Autodesk Fusion 360 part; units mm, degrees
note: some values were not read from the file. Chosen so that the rebuilt part matches the saved one: which bodies a step acts on; which pieces of a blend or face edit are solid. Set by a fixed rule: which sketch regions a step uses.
(part 2 of 2)
sketch "outline" plane through (0, 0, 0) normal (0, 0, 1) x (1, 0, 0)
  line L0 (16.3638, 40.64) -> (-16.3638, 40.64)
  line L1 (-40.64, 16.3638) -> (-40.64, -16.3638)
  line L2 (-16.3638, -40.64) -> (16.3638, -40.64)
  line L3 (40.64, -16.3638) -> (40.64, 16.3638)
  circle A0 centre (16.129, 37.719) radius 1.5
  circle A1 centre (-37.719, 16.129) radius 1.5
  circle A2 centre (-16.129, -37.719) radius 1.5
  circle A3 centre (37.719, -16.129) radius 1.5
  circle A4 centre (37.719, 16.129) radius 1.5
  circle A5 centre (-16.129, 37.719) radius 1.5
  circle A6 centre (-37.719, -16.129) radius 1.5
  circle A7 centre (16.129, -37.719) radius 1.5
  line L4 (-18.1316, 39.9078) -> (-39.9078, 18.1316)
  line L5 (-39.9078, -18.1316) -> (-18.1316, -39.9078)
  line L6 (18.1316, -39.9078) -> (39.9078, -18.1316)
  line L7 (39.9078, 18.1316) -> (18.1316, 39.9078)
  arc A8 (18.1316, 39.9078) -> (16.3638, 40.64) centre (16.3638, 38.14) ccw
  arc A9 (40.64, 16.3638) -> (39.9078, 18.1316) centre (38.14, 16.3638) ccw
  arc A10 (39.9078, -18.1316) -> (40.64, -16.3638) centre (38.14, -16.3638) ccw
  arc A11 (-40.64, -16.3638) -> (-39.9078, -18.1316) centre (-38.14, -16.3638) ccw
  arc A12 (-18.1316, -39.9078) -> (-16.3638, -40.64) centre (-16.3638, -38.14) ccw
  arc A13 (-16.3638, 40.64) -> (-18.1316, 39.9078) centre (-16.3638, 38.14) ccw
  arc A14 (-39.9078, 18.1316) -> (-40.64, 16.3638) centre (-38.14, 16.3638) ccw
  arc A15 (16.3638, -40.64) -> (18.1316, -39.9078) centre (16.3638, -38.14) ccw
  dimension "d2" = 40.64
  dimension "d3" = 3
  dimension "d4" = 16.129
  dimension "d5" = 37.719
  dimension "d7" = 360
  dimension "d8" = 3
  dimension "d9" = 16.129
  dimension "d10" = 37.719
  dimension "d12" = 360
  dimension "d14" = 2.5
  dimension "d15" = 2.5
  dimension "d16" = 2.5
  dimension "d17" = 2.5
  dimension "d18" = 2.5
  dimension "d19" = 2.5
  dimension "d20" = 2.5
  dimension "d23" = 2.5
  measures "d2" distance of origin L3
  measures "d3" diameter of A0
  measures "d4" distance of origin A0.centre
  measures "d5" distance of origin A0.centre
  measures "d8" diameter of A4
  measures "d9" distance of origin A4.centre
  measures "d10" distance of origin A4.centre
  measures "d14" radius of A8
  measures "d15" radius of A9
  measures "d16" radius of A10
  measures "d17" radius of A11
  measures "d18" radius of A12
  measures "d19" radius of A13
  measures "d20" radius of A14
  measures "d23" radius of A15
extrude "Extrude1" add sketch "outline" along normal blind 1.6 makes body 1
extrude "Extrude2" cut sketch "cpx crickit" along normal up to surface (1.6 mm away) contours A88 | A89 | A90 | A91 | A92 | A93 | A94 | A95 | A96 | A97 | A98 | A99 | A100 | A101 | A102 | A103 | A104 | A105 | A106 | A107 | A108 | A109 | A110 | A111 | A112 | A113 | A114 | A115 | A116 | A117 | A118 | A119 | A120 | A121 | A122 | A123 | A124 | A125 | A126 | A127 | A128 | A129 | A130 | A131 | A132 | A133 | A134 | A135 | A136 | A137 | A138 | A139 | A140 | A141 | A142 | A143 | A144 | A145 | A146 | A147 | A148 bodies 1
sketch "PCB" plane through (0, 0, 1.6) normal (0, 0, 1) x (-1, 0, 0)
  circle A0 centre (-26.1731, -21.2233) radius 0.635
  circle A1 centre (11.6332, -20.066) radius 1.5
  circle A2 centre (24.5963, -22.8001) radius 0.635
  circle A3 centre (19.2081, -24.5962) radius 0.635
  circle A4 centre (22.8002, -21.0041) radius 0.635
  circle A5 centre (33.528, 3.81) radius 0.635
  circle A6 centre (36.068, -1.27) radius 0.635
  circle A7 centre (33.528, -6.35) radius 0.635
  circle A8 centre (36.068, -8.89) radius 0.635
  circle A9 centre (30.988, -1.27) radius 0.635
  circle A10 centre (33.528, -8.89) radius 0.635
  circle A11 centre (-33.528, 0) radius 0.635
  circle A12 centre (-30.2288, 18.0312) radius 0.635
  circle A13 centre (-22.7949, 25.4651) radius 0.635
  circle A14 centre (24.8067, 29.5692) radius 1.5
  circle A15 centre (29.3787, 24.9972) radius 1.5
  circle A16 centre (-11.6332, 20.066) radius 1.5
  circle A17 centre (-27.7539, 20.5061) radius 0.635
  circle A18 centre (-33.528, 3.5) radius 0.635
  circle A19 centre (33.528, -1.27) radius 0.635
  circle A20 centre (36.068, 3.81) radius 0.635
  circle A21 centre (30.988, -6.35) radius 0.635
  circle A22 centre (30.988, 6.35) radius 0.635
  circle A23 centre (33.528, -3.81) radius 0.635
  circle A24 centre (36.068, -6.35) radius 0.635
  circle A25 centre (24.5963, -19.208) radius 0.635
  circle A26 centre (24.5963, -26.3922) radius 0.635
  circle A27 centre (22.8002, -24.5962) radius 0.635
  circle A28 centre (17.78, -14.859) radius 1.5
  circle A29 centre (-28.6479, -18.7485) radius 0.635
  circle A30 centre (-18.7485, -28.6479) radius 0.635
  circle A31 centre (21.844, -7.9248) radius 1.5
  circle A32 centre (21.0041, -22.8001) radius 0.635
  circle A33 centre (26.3923, -24.5962) radius 0.635
  circle A34 centre (26.3923, -21.0041) radius 0.635
  circle A35 centre (30.988, -3.81) radius 0.635
  circle A36 centre (30.988, 1.27) radius 0.635
  circle A37 centre (33.528, 8.89) radius 0.635
  circle A38 centre (36.068, 8.89) radius 0.635
  circle A39 centre (30.988, 8.89) radius 0.635
  circle A40 centre (36.068, 1.27) radius 0.635
  circle A41 centre (-33.528, -3.5) radius 0.635
  circle A42 centre (-21.844, 7.9248) radius 1.5
  circle A43 centre (-20.32, 27.94) radius 0.635
  circle A44 centre (20.1077, 34.2682) radius 1.5
  circle A45 centre (34.1412, 20.2982) radius 1.5
  circle A46 centre (-17.8451, 30.4149) radius 0.635
  circle A47 centre (-17.78, 14.859) radius 1.5
  circle A48 centre (-33.528, 7) radius 0.635
  circle A49 centre (-33.528, -7) radius 0.635
  circle A50 centre (30.988, -8.89) radius 0.635
  circle A51 centre (30.988, 3.81) radius 0.635
  circle A52 centre (33.528, 1.27) radius 0.635
  circle A53 centre (36.068, 6.35) radius 0.635
  circle A54 centre (33.528, 6.35) radius 0.635
  circle A55 centre (36.068, -3.81) radius 0.635
  circle A56 centre (22.8002, -28.1883) radius 0.635
  circle A57 centre (21.0041, -26.3922) radius 0.635
  circle A58 centre (28.1884, -22.8001) radius 0.635
  circle A59 centre (-21.2233, -26.1731) radius 0.635
  circle A60 centre (-23.6982, -23.6982) radius 0.635
  circle A61 centre (-16.129, -37.719) radius 1.5
  circle A62 centre (-16.129, 37.719) radius 1.5
  circle A63 centre (16.129, 37.719) radius 1.5
  circle A64 centre (-37.719, 16.129) radius 1.5
  circle A65 centre (16.129, -37.719) radius 1.5
  circle A66 centre (-37.719, -16.129) radius 1.5
  circle A67 centre (37.719, 16.129) radius 1.5
  circle A68 centre (37.719, -16.129) radius 1.5
  arc A69 (-16.3638, 40.64) -> (-18.1316, 39.9078) centre (-16.3638, 38.14) ccw
  line L0 (-18.1316, 39.9078) -> (-39.9078, 18.1316)
  arc A70 (-39.9078, 18.1316) -> (-40.64, 16.3638) centre (-38.14, 16.3638) ccw
  line L1 (-40.64, 16.3638) -> (-40.64, -16.3638)
  arc A71 (-40.64, -16.3638) -> (-39.9078, -18.1316) centre (-38.14, -16.3638) ccw
  line L2 (-39.9078, -18.1316) -> (-18.1316, -39.9078)
  arc A72 (-18.1316, -39.9078) -> (-16.3638, -40.64) centre (-16.3638, -38.14) ccw
  line L3 (-16.3638, -40.64) -> (16.3638, -40.64)
  arc A73 (16.3638, -40.64) -> (18.1316, -39.9078) centre (16.3638, -38.14) ccw
  line L4 (18.1316, -39.9078) -> (39.9078, -18.1316)
  arc A74 (39.9078, -18.1316) -> (40.64, -16.3638) centre (38.14, -16.3638) ccw
  line L5 (40.64, -16.3638) -> (40.64, 16.3638)
  arc A75 (40.64, 16.3638) -> (39.9078, 18.1316) centre (38.14, 16.3638) ccw
  line L6 (39.9078, 18.1316) -> (18.1316, 39.9078)
  arc A76 (18.1316, 39.9078) -> (16.3638, 40.64) centre (16.3638, 38.14) ccw
  line L7 (16.3638, 40.64) -> (-16.3638, 40.64)
  line L8 (37.518, -10.34) -> (29.538, -10.34)
  line L9 (29.538, -10.34) -> (29.538, 10.34)
  line L10 (29.538, 10.34) -> (37.518, 10.34)
  line L11 (37.518, 10.34) -> (37.518, -10.34)
  line L12 (22.8002, -29.9844) -> (29.9844, -22.8001)
  line L13 (29.9844, -22.8001) -> (24.5963, -17.412)
  line L14 (24.5963, -17.412) -> (17.412, -24.5962)
  line L15 (17.412, -24.5962) -> (22.8002, -29.9844)
  line L16 (24.5963, -28.1883) -> (19.2081, -22.8001)
  line L17 (26.3923, -26.3922) -> (21.0041, -21.0041)
  line L18 (28.1884, -24.5962) -> (22.8002, -19.208)
  line L19 (-3.8, 40.64) -> (3.8, 40.64)
  line L20 (3.8, 40.64) -> (3.8, 35.04)
  line L21 (3.8, 35.04) -> (-3.8, 35.04)
  line L22 (-3.8, 35.04) -> (-3.8, 40.64)
  line L23 (-3.8, 40.64) -> (3.8, 35.04) construction
  line L24 (3.8, 40.64) -> (-3.8, 35.04) construction
  line L25 (0, 37.84) -> (0, 40.64) construction
  line L26 (6.505, 39.4055) -> (10.005, 39.4055)
  line L27 (10.005, 39.4055) -> (10.005, 35.9055)
  line L28 (10.005, 35.9055) -> (6.505, 35.9055)
  line L29 (6.505, 35.9055) -> (6.505, 39.4055)
  line L30 (6.505, 39.4055) -> (10.005, 35.9055) construction
  line L31 (10.005, 39.4055) -> (6.505, 35.9055) construction
  line L32 (3.865, -29.74) -> (-5.135, -29.74)
  line L33 (-5.135, -29.74) -> (-5.135, -44.14)
  line L34 (-5.135, -44.14) -> (3.865, -44.14)
  line L35 (3.865, -44.14) -> (3.865, -29.74)
  line L36 (3.865, -29.74) -> (-5.135, -44.14) construction
  line L37 (-5.135, -29.74) -> (3.865, -44.14) construction
  line L38 (-12.017, -33.195) -> (-6.017, -33.195)
  line L39 (-6.017, -33.195) -> (-6.017, -39.195)
  line L40 (-6.017, -39.195) -> (-12.017, -39.195)
  line L41 (-12.017, -39.195) -> (-12.017, -33.195)
  line L42 (-12.017, -33.195) -> (-6.017, -39.195) construction
  line L43 (-6.017, -33.195) -> (-12.017, -39.195) construction
  circle A77 centre (-9.017, -36.195) radius 1.5
  line L44 (8.029, -31.679) -> (11.529, -31.679)
  line L45 (11.529, -31.679) -> (11.529, -38.679)
  line L46 (11.529, -38.679) -> (8.029, -38.679)
  line L47 (8.029, -38.679) -> (8.029, -31.679)
  line L48 (8.029, -31.679) -> (11.529, -38.679) construction
  line L49 (11.529, -31.679) -> (8.029, -38.679) construction
  line L50 (15.6765, -27.19) -> (14.6765, -27.19)
  line L51 (14.6765, -27.19) -> (14.6765, -28.69)
  line L52 (14.6765, -28.69) -> (15.6765, -28.69)
  line L53 (15.6765, -28.69) -> (15.6765, -27.19)
  line L54 (15.6765, -27.19) -> (14.6765, -28.69) construction
  line L55 (14.6765, -27.19) -> (15.6765, -28.69) construction
  line L56 (13.2635, -27.19) -> (12.2635, -27.19)
  line L57 (12.2635, -27.19) -> (12.2635, -28.69)
  line L58 (12.2635, -28.69) -> (13.2635, -28.69)
  line L59 (13.2635, -28.69) -> (13.2635, -27.19)
  line L60 (13.2635, -27.19) -> (12.2635, -28.69) construction
  line L61 (12.2635, -27.19) -> (13.2635, -28.69) construction
  line L62 (31.369, -14.7236) -> (35.1874, -18.542)
  line L63 (35.1874, -18.542) -> (31.369, -22.3604)
  line L64 (31.369, -22.3604) -> (27.5506, -18.542)
  line L65 (27.5506, -18.542) -> (31.369, -14.7236)
  line L66 (31.369, -14.7236) -> (31.369, -22.3604) construction
  line L67 (35.1874, -18.542) -> (27.5506, -18.542) construction
  circle A78 centre (31.369, -18.542) radius 2.5
  line L68 (-34.577, -9.746) -> (-29.177, -9.746)
  line L69 (-29.177, -9.746) -> (-29.177, -15.146)
  line L70 (-29.177, -15.146) -> (-34.577, -15.146)
  line L71 (-34.577, -15.146) -> (-34.577, -9.746)
  line L72 (-34.577, -9.746) -> (-29.177, -15.146) construction
  line L73 (-29.177, -9.746) -> (-34.577, -15.146) construction
  circle A79 centre (-31.877, -12.446) radius 2.5
  line L74 (-30.128, -9) -> (-36.928, -9)
  line L75 (-36.928, -9) -> (-36.928, 9)
  line L76 (-36.928, 9) -> (-30.128, 9)
  line L77 (-30.128, 9) -> (-30.128, -9)
  line L78 (-19.7384, -32.4663) -> (-32.4664, -19.7384)
  line L79 (-32.4664, -19.7384) -> (-27.658, -14.93)
  line L80 (-27.658, -14.93) -> (-14.9301, -27.658)
  line L81 (-14.9301, -27.658) -> (-19.7384, -32.4663)
  line L82 (-21.805, 21.6467) -> (-26.6133, 26.455)
  line L83 (-26.6133, 26.455) -> (-18.8351, 34.2332)
  line L84 (-18.8351, 34.2332) -> (-14.0268, 29.4249)
  line L85 (-14.0268, 29.4249) -> (-21.805, 21.6467)
  line L86 (-24.2091, 24.0509) -> (-16.4309, 31.8291) construction
  line L87 (-29.2389, 14.2128) -> (-23.9355, 19.5161)
  line L88 (-23.9355, 19.5161) -> (-28.7439, 24.3245)
  line L89 (-28.7439, 24.3245) -> (-34.0472, 19.0211)
  line L90 (-34.0472, 19.0211) -> (-29.2389, 14.2128)
  circle A80 centre (-20.141, 20.194) radius 1.5
  line L91 (-3.5, 29.154) -> (3.5, 29.154)
  line L92 (3.5, 29.154) -> (3.5, 22.154)
  line L93 (3.5, 22.154) -> (-3.5, 22.154)
  line L94 (-3.5, 22.154) -> (-3.5, 29.154)
  line L95 (-3.5, 29.154) -> (3.5, 22.154) construction
  line L96 (3.5, 29.154) -> (-3.5, 22.154) construction
  line L97 (-18.456, 4.659) -> (-14.056, 4.659)
  line L98 (-14.056, 4.659) -> (-14.056, -0.341)
  line L99 (-14.056, -0.341) -> (-18.456, -0.341)
  line L100 (-18.456, -0.341) -> (-18.456, 4.659)
  line L101 (-18.456, 4.659) -> (-14.056, -0.341) construction
  line L102 (-14.056, 4.659) -> (-18.456, -0.341) construction
  line L103 (-17.3046, -9.9859) -> (-14.4762, -7.1575)
  line L104 (-14.4762, -7.1575) -> (-7.4051, -14.2286)
  line L105 (-7.4051, -14.2286) -> (-10.2336, -17.057)
  line L106 (-10.2336, -17.057) -> (-17.3046, -9.9859)
  line L107 (-17.3046, -9.9859) -> (-7.4051, -14.2286) construction
  line L108 (-14.4762, -7.1575) -> (-10.2336, -17.057) construction
  point P0 (0, 37.84)
  point P1 (8.255, 37.6555)
  point P2 (-0.635, -36.94)
  point P3 (-9.017, -36.195)
  point P4 (9.779, -35.179)
  point P5 (15.1765, -27.94)
  point P6 (12.7635, -27.94)
  point P7 (31.369, -18.542)
  point P8 (-31.877, -12.446)
  point P9 (0, 25.654)
  point P10 (-16.256, 2.159)
  point P11 (-12.3549, -12.1073)
  dimension "d61" = 1.45
  dimension "d62" = 1.45
  dimension "d63" = 1.45
  dimension "d64" = 1.45
  dimension "d81" = 90
  dimension "d82" = 90
  dimension "d83" = 1.27
  dimension "d84" = 1.27
  dimension "d88" = 2.54
  dimension "d89" = 0
  dimension "d90" = 1.27
  dimension "d91" = 1.27
  dimension "d92" = 1.27
  dimension "d110" = 7.6
  dimension "d111" = 5.6
  dimension "d117" = 3.5
  dimension "d118" = 3.5
  dimension "d119" = 8.255
  dimension "d120" = 37.6555
  dimension "d126" = 9
  dimension "d127" = 14.4
  dimension "d128" = 0.635
  dimension "d129" = 3.5
  dimension "d147" = 6
  dimension "d148" = 6
  dimension "d149" = 9.017
  dimension "d150" = 36.195
  dimension "d151" = 3
  dimension "d157" = 7
  dimension "d158" = 3.5
  dimension "d159" = 9.779
  dimension "d160" = 35.179
  dimension "d170" = 1.5
  dimension "d171" = 1
  dimension "d172" = 15.1765
  dimension "d173" = 27.94
  dimension "d174" = 1.5
  dimension "d175" = 1
  dimension "d176" = 12.7635
  dimension "d179" = 5.4
  dimension "d180" = 5.4
  dimension "d181" = 31.369
  dimension "d182" = 18.542
  dimension "d183" = 5
  dimension "d190" = 5.4
  dimension "d191" = 5.4
  dimension "d192" = 5
  dimension "d193" = 31.877
  dimension "d194" = 12.446
  dimension "d201" = 3.4
  dimension "d202" = 3.4
  dimension "d203" = 2
  dimension "d204" = 2
  dimension "d239" = 2
  dimension "d241" = 90
  dimension "d242" = 90
  dimension "d243" = 3.4
  dimension "d244" = 18
  dimension "d277" = 3.4
  dimension "d278" = 3.4
  dimension "d279" = 2
  dimension "d282" = 11
  dimension "d283" = 2
  dimension "d284" = 3.4
  dimension "d285" = 3.4
  dimension "d286" = 7.5
  dimension "d338" = 3
  dimension "d339" = 20.194
  dimension "d340" = 20.141
  dimension "d349" = 7
  dimension "d350" = 7
  dimension "d351" = 25.654
  dimension "d354" = 4.4
  dimension "d355" = 5
  dimension "d356" = 16.256
  dimension "d360" = 2.159
  dimension "d361" = 10
  dimension "d362" = 4
  dimension "d363" = 12.3549
  dimension "d364" = 12.1073
  measures "d61" distance of A8.centre L11
  measures "d62" distance of A8.centre L8
  measures "d63" distance of A50.centre L9
  measures "d64" distance of A39.centre L10
  measures "d81" angle of L12 L13
  measures "d82" angle of L13 L14
  measures "d83" distance of A58.centre L13
  measures "d84" distance of A58.centre L12
  measures "d90" distance of A56.centre L15
  measures "d91" distance of A57.centre L16
  measures "d92" distance of A3.centre L14
  measures "d110" distance of L20.end L21.end
  measures "d111" distance of L19.end L20.end
  measures "d117" distance of L27.end L28.end
  measures "d118" distance of L26.end L27.end
  measures "d119" distance of origin P1
  measures "d120" distance of origin P1
  measures "d126" distance of L33.end L34.end
  measures "d127" distance of L32.end L33.end
  measures "d128" distance of origin P2
  measures "d129" distance of L3 L34
  measures "d147" distance of L39.end L40.end
  measures "d148" distance of L38.end L39.end
  measures "d149" distance of origin P3
  measures "d150" distance of origin P3
  measures "d151" diameter of A77
  measures "d157" distance of L44.end L45.end
  measures "d158" distance of L45.end L46.end
  measures "d159" distance of origin P4
  measures "d160" distance of origin P4
  measures "d170" distance of L50.end L51.end
  measures "d171" distance of L51.end L52.end
  measures "d172" distance of origin P5
  measures "d173" distance of origin P5
  measures "d174" distance of L56.end L57.end
  measures "d175" distance of L57.end L58.end
  measures "d176" distance of origin P6
  measures "d179" distance of L62.end L63.end
  measures "d180" distance of L63.end L64.end
  measures "d181" distance of origin P7
  measures "d182" distance of origin P7
  measures "d183" diameter of A78
  measures "d190" distance of L69.end L70.end
  measures "d191" distance of L68.end L69.end
  measures "d192" diameter of A79
  measures "d193" distance of origin P8
  measures "d194" distance of origin P8
  measures "d201" distance of A48.centre L75
  measures "d202" distance of A48.centre L77
  measures "d203" distance of A48.centre L76
  measures "d204" distance of A49.centre L74
  measures "d239" distance of A30.centre L81
  measures "d241" angle of L78 L81
  measures "d242" angle of L79 L80
  measures "d243" distance of A30.centre L80
  measures "d244" distance of L78.start L78.end
  measures "d277" distance of A13.centre L83
  measures "d278" distance of A13.centre L85
  measures "d279" distance of A13.centre L82
  measures "d282" distance of L86.start L86.end
  measures "d283" distance of A12.centre L90
  measures "d284" distance of A12.centre L87
  measures "d285" distance of A12.centre L89
  measures "d286" distance of L87.start L87.end
  measures "d338" diameter of A80
  measures "d339" distance of origin A80.centre
  measures "d340" distance of origin A80.centre
  measures "d349" distance of L92.end L93.end
  measures "d350" distance of L91.end L92.end
  measures "d351" distance of origin P9
  measures "d354" distance of L98.end L99.end
  measures "d355" distance of L97.end L98.end
  measures "d356" distance of origin P10
  measures "d360" distance of origin P10
  measures "d361" distance of L103.end L104.end
  measures "d362" distance of L104.end L105.end
  measures "d363" distance of origin P11
  measures "d364" distance of origin P11
extrude "Extrude8" add sketch "PCB" along normal blind 1 separate body contours L26 L27 L28 L29 makes body 2
extrude "Extrude3" add sketch "PCB" along normal blind 8.6 separate body contours A5 | A6 | A7 | A8 | A9 | A10 | A19 | A20 | A21 | A22 | A23 | A24 | A35 | A36 | A37 | A38 | A39 | A40 | A50 | A51 | A52 | A53 | A54 | A55 | L8 L9 L10 L11 makes body 3
sketch "sio block" plane through (0, 0, 10.2) normal (0, 0, 1) x (-1, 0, 0)
  line L0 (37.518, 10.34) -> (29.538, 10.34)
  line L1 (29.538, 10.34) -> (29.538, -10.34)
  line L2 (29.538, -10.34) -> (37.518, -10.34)
  line L3 (37.518, -10.34) -> (37.518, 10.34)
  line L4 (35.768, -8.59) -> (36.368, -8.59)
  line L5 (36.368, -8.59) -> (36.368, -9.19)
  line L6 (36.368, -9.19) -> (35.768, -9.19)
  line L7 (35.768, -9.19) -> (35.768, -8.59)
  line L8 (35.768, -8.59) -> (36.368, -9.19) construction
  line L9 (36.368, -8.59) -> (35.768, -9.19) construction
  line L10 (33.828, -9.19) -> (33.228, -9.19)
  line L11 (33.228, -9.19) -> (33.228, -8.59)
  line L12 (33.228, -8.59) -> (33.828, -8.59)
  line L13 (33.828, -8.59) -> (33.828, -9.19)
  line L14 (31.288, -9.19) -> (30.688, -9.19)
  line L15 (30.688, -9.19) -> (30.688, -8.59)
  line L16 (30.688, -8.59) -> (31.288, -8.59)
  line L17 (31.288, -8.59) -> (31.288, -9.19)
  line L18 (36.368, -6.65) -> (35.768, -6.65)
  line L19 (35.768, -6.65) -> (35.768, -6.05)
  line L20 (35.768, -6.05) -> (36.368, -6.05)
  line L21 (36.368, -6.05) -> (36.368, -6.65)
  line L22 (33.828, -6.65) -> (33.228, -6.65)
  line L23 (33.228, -6.65) -> (33.228, -6.05)
  line L24 (33.228, -6.05) -> (33.828, -6.05)
  line L25 (33.828, -6.05) -> (33.828, -6.65)
  line L26 (31.288, -6.65) -> (30.688, -6.65)
  line L27 (30.688, -6.65) -> (30.688, -6.05)
  line L28 (30.688, -6.05) -> (31.288, -6.05)
  line L29 (31.288, -6.05) -> (31.288, -6.65)
  line L30 (36.368, -4.11) -> (35.768, -4.11)
  line L31 (35.768, -4.11) -> (35.768, -3.51)
  line L32 (35.768, -3.51) -> (36.368, -3.51)
  line L33 (36.368, -3.51) -> (36.368, -4.11)
  line L34 (33.828, -4.11) -> (33.228, -4.11)
  line L35 (33.228, -4.11) -> (33.228, -3.51)
  line L36 (33.228, -3.51) -> (33.828, -3.51)
  line L37 (33.828, -3.51) -> (33.828, -4.11)
  line L38 (31.288, -4.11) -> (30.688, -4.11)
  line L39 (30.688, -4.11) -> (30.688, -3.51)
  line L40 (30.688, -3.51) -> (31.288, -3.51)
  line L41 (31.288, -3.51) -> (31.288, -4.11)
  line L42 (36.368, -1.57) -> (35.768, -1.57)
  line L43 (35.768, -1.57) -> (35.768, -0.97)
  line L44 (35.768, -0.97) -> (36.368, -0.97)
  line L45 (36.368, -0.97) -> (36.368, -1.57)
  line L46 (33.828, -1.57) -> (33.228, -1.57)
  line L47 (33.228, -1.57) -> (33.228, -0.97)
  line L48 (33.228, -0.97) -> (33.828, -0.97)
  line L49 (33.828, -0.97) -> (33.828, -1.57)
  line L50 (31.288, -1.57) -> (30.688, -1.57)
  line L51 (30.688, -1.57) -> (30.688, -0.97)
  line L52 (30.688, -0.97) -> (31.288, -0.97)
  line L53 (31.288, -0.97) -> (31.288, -1.57)
  line L54 (36.368, 0.97) -> (35.768, 0.97)
  line L55 (35.768, 0.97) -> (35.768, 1.57)
  line L56 (35.768, 1.57) -> (36.368, 1.57)
  line L57 (36.368, 1.57) -> (36.368, 0.97)
  line L58 (33.828, 0.97) -> (33.228, 0.97)
  line L59 (33.228, 0.97) -> (33.228, 1.57)
  line L60 (33.228, 1.57) -> (33.828, 1.57)
  line L61 (33.828, 1.57) -> (33.828, 0.97)
  line L62 (31.288, 0.97) -> (30.688, 0.97)
  line L63 (30.688, 0.97) -> (30.688, 1.57)
  line L64 (30.688, 1.57) -> (31.288, 1.57)
  line L65 (31.288, 1.57) -> (31.288, 0.97)
  line L66 (36.368, 3.51) -> (35.768, 3.51)
  line L67 (35.768, 3.51) -> (35.768, 4.11)
  line L68 (35.768, 4.11) -> (36.368, 4.11)
  line L69 (36.368, 4.11) -> (36.368, 3.51)
  line L70 (33.828, 3.51) -> (33.228, 3.51)
  line L71 (33.228, 3.51) -> (33.228, 4.11)
  line L72 (33.228, 4.11) -> (33.828, 4.11)
  line L73 (33.828, 4.11) -> (33.828, 3.51)
  line L74 (31.288, 3.51) -> (30.688, 3.51)
  line L75 (30.688, 3.51) -> (30.688, 4.11)
  line L76 (30.688, 4.11) -> (31.288, 4.11)
  line L77 (31.288, 4.11) -> (31.288, 3.51)
  line L78 (36.368, 6.05) -> (35.768, 6.05)
  line L79 (35.768, 6.05) -> (35.768, 6.65)
  line L80 (35.768, 6.65) -> (36.368, 6.65)
  line L81 (36.368, 6.65) -> (36.368, 6.05)
  line L82 (33.828, 6.05) -> (33.228, 6.05)
  line L83 (33.228, 6.05) -> (33.228, 6.65)
  line L84 (33.228, 6.65) -> (33.828, 6.65)
  line L85 (33.828, 6.65) -> (33.828, 6.05)
  line L86 (31.288, 6.05) -> (30.688, 6.05)
  line L87 (30.688, 6.05) -> (30.688, 6.65)
  line L88 (30.688, 6.65) -> (31.288, 6.65)
  line L89 (31.288, 6.65) -> (31.288, 6.05)
  line L90 (36.368, 8.59) -> (35.768, 8.59)
  line L91 (35.768, 8.59) -> (35.768, 9.19)
  line L92 (35.768, 9.19) -> (36.368, 9.19)
  line L93 (36.368, 9.19) -> (36.368, 8.59)
  line L94 (33.828, 8.59) -> (33.228, 8.59)
  line L95 (33.228, 8.59) -> (33.228, 9.19)
  line L96 (33.228, 9.19) -> (33.828, 9.19)
  line L97 (33.828, 9.19) -> (33.828, 8.59)
  line L98 (31.288, 8.59) -> (30.688, 8.59)
  line L99 (30.688, 8.59) -> (30.688, 9.19)
  line L100 (30.688, 9.19) -> (31.288, 9.19)
  line L101 (31.288, 9.19) -> (31.288, 8.59)
  point P0 (36.068, -8.89)
  dimension "d67" = 0.6
  dimension "d68" = 0.6
  dimension "d69" = 1.45
  dimension "d70" = 1.45
  dimension "d73" = -2.54
  dimension "d74" = 2.54
  measures "d67" distance of L4.end L5.end
  measures "d68" distance of L5.end L6.end
  measures "d69" distance of L3 P0
  measures "d70" distance of L2 P0
extrude "Extrude4" cut sketch "sio block" against normal up to surface (8.6 mm away) contours L4 L5 L6 L7 | L10 L11 L12 L13 | L14 L15 L16 L17 | L18 L19 L20 L21 | L22 L23 L24 L25 | L26 L27 L28 L29 | L30 L31 L32 L33 | L34 L35 L36 L37 | L38 L39 L40 L41 | L42 L43 L44 L45 | L46 L47 L48 L49 | L50 L51 L52 L53 | L54 L55 L56 L57 | L58 L59 L60 L61 | L62 L63 L64 L65 | L66 L67 L68 L69 | L70 L71 L72 L73 | L74 L75 L76 L77 | L78 L79 L80 L81 | L82 L83 L84 L85 | L86 L87 L88 L89 | L90 L91 L92 L93 | L94 L95 L96 L97 | L98 L99 L100 L101 bodies 3
chamfer "Chamfer1" distance 0.2 angle 45 96 edges at (-30.988, 8.59, 10.2) (-30.688, 8.89, 10.2) (-30.988, 9.19, 10.2) (-31.288, 8.89, 10.2) (-33.828, 8.89, 10.2) (-33.528, 9.19, 10.2) (-33.228, 8.89, 10.2) (-33.528, 8.59, 10.2) (-35.768, 8.89, 10.2) (-36.068, 8.59, 10.2) (-36.368, 8.89, 10.2) (-36.068, 9.19, 10.2) (-36.068, 6.05, 10.2) (-36.368, 6.35, 10.2) (-36.068, 6.65, 10.2) (-35.768, 6.35, 10.2) (-33.828, 6.35, 10.2) (-33.528, 6.65, 10.2) (-33.228, 6.35, 10.2) (-33.528, 6.05, 10.2) (-31.288, 6.35, 10.2) (-30.988, 6.05, 10.2) (-30.688, 6.35, 10.2) (-30.988, 6.65, 10.2) (-36.068, 4.11, 10.2) (-36.368, 3.81, 10.2) (-36.068, 3.51, 10.2) (-35.768, 3.81, 10.2) (-33.828, 1.27, 10.2) (-33.528, 1.57, 10.2) (-33.228, 1.27, 10.2) (-33.528, 0.97, 10.2) (-31.288, -1.27, 10.2) (-30.988, -0.97, 10.2) (-30.688, -1.27, 10.2) (-30.988, -1.57, 10.2) (-33.228, -1.27, 10.2) (-33.528, -0.97, 10.2) (-33.828, -1.27, 10.2) (-33.528, -1.57, 10.2) (-36.068, -0.97, 10.2) (-35.768, -1.27, 10.2) (-36.368, -1.27, 10.2) (-36.068, -1.57, 10.2) (-35.768, 1.27, 10.2) (-36.068, 0.97, 10.2) (-36.368, 1.27, 10.2) (-36.068, 1.57, 10.2) (-33.228, 3.81, 10.2) (-33.828, 3.81, 10.2) (-33.528, 4.11, 10.2) (-33.528, 3.51, 10.2) (-30.988, 1.57, 10.2) (-31.288, 1.27, 10.2) (-30.988, 0.97, 10.2) (-30.688, 1.27, 10.2) (-30.988, 3.51, 10.2) (-31.288, 3.81, 10.2) (-30.988, 4.11, 10.2) (-30.688, 3.81, 10.2) (-36.368, -3.81, 10.2) (-35.768, -3.81, 10.2) (-36.068, -3.51, 10.2) (-36.068, -4.11, 10.2) (-36.068, -6.05, 10.2) (-36.368, -6.35, 10.2) (-36.068, -6.65, 10.2) (-35.768, -6.35, 10.2) (-30.988, -8.59, 10.2) (-31.288, -8.89, 10.2) (-30.988, -9.19, 10.2) (-30.688, -8.89, 10.2) (-33.228, -8.89, 10.2) (-33.528, -9.19, 10.2) (-33.828, -8.89, 10.2) (-33.528, -8.59, 10.2) (-35.768, -8.89, 10.2) (-36.068, -8.59, 10.2) (-36.068, -9.19, 10.2) (-36.368, -8.89, 10.2) (-33.828, -6.35, 10.2) (-33.528, -6.65, 10.2) (-33.228, -6.35, 10.2) (-33.528, -6.05, 10.2) (-31.288, -6.35, 10.2) (-30.988, -6.65, 10.2) (-30.688, -6.35, 10.2) (-30.988, -6.05, 10.2) (-30.988, -4.11, 10.2) (-31.288, -3.81, 10.2) (-33.228, -3.81, 10.2) (-33.528, -4.11, 10.2) (-33.828, -3.81, 10.2) (-33.528, -3.51, 10.2) (-30.988, -3.51, 10.2) (-30.688, -3.81, 10.2) on bodies 3
extrude "Extrude5" add sketch "PCB" along normal blind 2.2 separate body contours A3 | A56 | A57 | L12 L14 L15 L16 makes body 4
chamfer "Chamfer3" distance 0.4 angle 45 4 edges at (-24.5963, 28.1883, 2.7) (-22.8002, 29.9844, 2.7) (-17.412, 24.5962, 2.7) (-19.2081, 22.8001, 2.7) on bodies 4
pattern_linear "R-Pattern1" count 4 spacing 2.54 along (-0.707107, -0.707107, 0) of bodies 4 makes body 5 at (-23.3046, 25.6993, 1.6) makes body 6 at (-25.1007, 23.9032, 1.6) makes body 7 at (-26.8967, 22.1072, 1.6)
combine "Combine1" operation add target body 7 tool bodies 4 5 6
sketch "servo block" plane through (0, 0, 3.8) normal (0, 0, 1) x (-1, 0, 0)
  line L0 (19.4909, -23.083) -> (18.9253, -23.083)
  line L1 (18.9253, -23.083) -> (17.6949, -24.3134)
  line L2 (17.6949, -24.3134) -> (17.6949, -24.879)
  line L3 (17.6949, -24.879) -> (22.5174, -29.7015)
  line L4 (22.5174, -29.7015) -> (23.083, -29.7015)
  line L5 (23.083, -29.7015) -> (24.3134, -28.4711)
  line L6 (24.3134, -28.4711) -> (24.3134, -27.9055)
  curve K0
  line L7 (24.8791, -27.9055) -> (26.1095, -26.6751)
  line L8 (26.1095, -26.6751) -> (26.1095, -26.1094)
  line L9 (26.1095, -26.1094) -> (26.6751, -26.1094)
  line L10 (26.6751, -26.1094) -> (27.9055, -24.879)
  line L11 (27.9055, -24.879) -> (27.9055, -24.3134)
  line L12 (27.9055, -24.3134) -> (28.4712, -24.3134)
  line L13 (28.4712, -24.3134) -> (29.7016, -23.083)
  line L14 (29.7016, -23.083) -> (29.7016, -22.5173)
  line L15 (29.7016, -22.5173) -> (24.8791, -17.6948)
  line L16 (24.8791, -17.6948) -> (24.3134, -17.6948)
  line L17 (24.3134, -17.6948) -> (23.083, -18.9252)
  line L18 (23.083, -18.9252) -> (23.083, -19.4909)
  line L19 (23.083, -19.4909) -> (22.5174, -19.4909)
  line L20 (22.5174, -19.4909) -> (21.287, -20.7213)
  line L21 (21.287, -20.7213) -> (21.287, -21.2869)
  line L22 (21.287, -21.2869) -> (20.7213, -21.2869)
  line L23 (20.7213, -21.2869) -> (19.4909, -22.5173)
  line L24 (19.4909, -22.5173) -> (19.4909, -23.083)
  line L25 (22.8002, -27.764) -> (22.3759, -28.1883)
  line L26 (22.3759, -28.1883) -> (22.8002, -28.6126)
  line L27 (22.8002, -28.6126) -> (23.2245, -28.1883)
  line L28 (23.2245, -28.1883) -> (22.8002, -27.764)
  line L29 (22.8002, -27.764) -> (22.8002, -28.6126) construction
  line L30 (22.3759, -28.1883) -> (23.2245, -28.1883) construction
  point P0 (22.8002, -28.1883)
  dimension "d100" = 0.6
  dimension "d101" = 0.6
  dimension "d102" = 1.27
  dimension "d103" = 1.27
  measures "d100" distance of L26.end L27.end
  measures "d101" distance of L25.end L26.end
  measures "d102" distance of L3 P0
  measures "d103" distance of L5 P0
extrude "Extrude6" add sketch "servo block" along normal blind 6 separate body makes body 8
pattern_linear "R-Pattern2" count 3 spacing 2.54 along (0.707107, -0.707107, 0) count 4 spacing 2.54 along (-0.707107, -0.707107, 0) of "Extrude6" makes body 9 at (-20.7213, 26.5337, 5.8) makes body 10 at (-18.9253, 24.7376, 5.8) makes body 11 at (-24.3134, 26.5337, 5.8) makes body 12 at (-22.6588, 24.3134, 5.8) makes body 13 at (-20.7213, 22.9416, 5.8) makes body 14 at (-26.1095, 24.7376, 5.8) makes body 15 at (-24.3134, 22.9416, 5.8) makes body 16 at (-22.5174, 21.1455, 5.8) makes body 17 at (-27.9055, 22.9416, 5.8) makes body 18 at (-26.1095, 21.1455, 5.8) makes body 19 at (-24.3134, 19.3495, 5.8)
copy_body "Body->Comp1" bodies 7 removing the originals makes body 20 in component "servo block"
copy_body "CutPasteBodies1" bodies 19 18 16 8 12 10 9 14 13 17 11 15 removing the originals makes body 21 makes body 22 makes body 23 makes body 24 makes body 25 makes body 26 makes body 27 makes body 28 makes body 29 makes body 30 makes body 31 makes body 32 in component "servo block"
extrude "Extrude7" add sketch "PCB" along normal blind 3 separate body contours L7 L19 L20 L21 L22 makes body 33
chamfer "Chamfer4" distance 1 angle 45 2 edges at (-3.8, -37.84, 1.6) (3.8, -37.84, 1.6) on bodies 33
shell "Shell1" thickness 0.4 removed faces 1 at (-0.9333, -40.64, 3.6) on bodies 33
sketch "neopixel" plane through (0, 0, 2.6) normal (0, 0, 1) x (-1, 0, 0)
  line L0 (6.505, 35.9055) -> (10.005, 35.9055)
  line L1 (10.005, 35.9055) -> (10.005, 39.4055)
  line L2 (10.005, 39.4055) -> (6.505, 39.4055)
  line L3 (6.505, 39.4055) -> (6.505, 35.9055)
  circle A0 centre (8.255, 37.6555) radius 1.5
  dimension "d123" = 3
  measures "d123" diameter of A0
extrude "Extrude9" cut sketch "neopixel" against normal blind 0.2 contours A0 bodies 2
extrude "Extrude10" add sketch "PCB" along normal blind 11 separate body contours L3 L33 L34 L35 makes body 34
extrude "Extrude11" add sketch "PCB" along normal blind 10.5 separate body contours L3 L32 L33 L35 makes body 35
fillet "Fillet1" radius 4.5 2 edges at (5.135, 35.19, 12.1) (-3.865, 35.19, 12.1) on bodies 35
sketch "dc jack" plane through (0, 44.14, 0) normal (0, 1, 0) x (-1, 0, 0)
  line L0 (-5.135, 1.6) -> (3.865, 1.6)
  line L1 (3.865, 1.6) -> (3.865, 12.6)
  line L2 (3.865, 12.6) -> (-5.135, 12.6)
  line L3 (-5.135, 12.6) -> (-5.135, 1.6)
  circle A0 centre (-0.635, 8.1) radius 3.25
  circle A1 centre (-0.635, 8.1) radius 1
  dimension "d136" = 6.5
  dimension "d138" = 2
  dimension "d146" = 6.5
  measures "d136" diameter of A0
  measures "d138" diameter of A1
  measures "d146" distance of L0 A0.centre
combine "Combine2" operation add target body 34 tool bodies 35
extrude "Extrude12" cut sketch "dc jack" against normal blind 9 contours A0 | A1 bodies 34
extrude "Extrude13" add sketch "dc jack" along normal blind 8 from surface at -9 contours A1 bodies 34
fillet "Fillet2" radius 1 1 edges at (1.5673, 43.14, 7.7384) on bodies 34
fillet "Fillet3" radius 0.4 4 edges at (5.135, 42.39, 12.6) (-3.865, 42.39, 12.6) (-3.865, 36.94, 1.6) (5.135, 36.94, 1.6) on bodies 34
extrude "Extrude14" add sketch "PCB" along normal blind 2 separate body contours L38 L39 L40 L41 | A77 makes body 36
extrude "Extrude15" add sketch "PCB" along normal blind 1 from surface at 2 contours A77 bodies 36
extrude "Extrude16" add sketch "PCB" along normal blind 1.6 separate body contours L44 L45 L46 L47 makes body 37
sketch "switch" plane through (0, 0, 3.2) normal (0, 0, 1) x (-1, 0, 0)
  line L0 (8.029, -38.679) -> (11.529, -38.679)
  line L1 (11.529, -38.679) -> (11.529, -31.679)
  line L2 (11.529, -31.679) -> (8.029, -31.679)
  line L3 (8.029, -31.679) -> (8.029, -38.679)
  line L4 (9.229, -36.679) -> (8.029, -36.679)
  line L5 (8.029, -36.679) -> (8.029, -33.679)
  line L6 (8.029, -33.679) -> (9.229, -33.679)
  line L7 (9.229, -33.679) -> (9.229, -36.679)
  line L8 (9.229, -35.179) -> (8.029, -35.179)
  dimension "d163" = 1.2
  dimension "d164" = 3
  measures "d163" distance of L4.start L4.end
  measures "d164" distance of L4.start L6.end
extrude "Extrude17" cut sketch "switch" against normal blind 0.2 contours L3 L4 L5 L7 L8 | L3 L5 L6 L7 L8 bodies 37
extrude "Extrude18" add sketch "switch" along normal blind 1.5 from surface at -0.2 contours L3 L4 L5 L7 L8 bodies 37
extrude "Extrude19" add sketch "PCB" along normal blind 1 separate body contours L50 L51 L52 L53 | L56 L57 L58 L59 makes body 38 at (-12.2635, 27.69, 1.9333) makes body 39 at (-14.6765, 27.69, 1.9333)
extrude "Extrude20" add sketch "PCB" along normal blind 0.4 separate body contours L62 L63 L64 L65 | A78 makes body 40
chamfer "Chamfer5" distance 1 angle 45 2 edges at (-31.369, 14.7236, 1.8) (-27.5506, 18.542, 1.8) on bodies 40
extrude "Extrude21" add sketch "PCB" along normal blind 5.4 contours A78 bodies 40
fillet "Fillet4" radius 0.5 1 edges at (-29.0382, 19.446, 7) on bodies 40
extrude "Extrude22" add sketch "PCB" along normal blind 0.4 separate body contours L68 L69 L70 L71 | A79 makes body 41
chamfer "Chamfer6" distance 1 angle 45 2 edges at (29.177, 9.746, 1.8) (29.177, 15.146, 1.8) on bodies 41
extrude "Extrude23" add sketch "PCB" along normal blind 5.4 contours A79 bodies 41
fillet "Fillet5" radius 0.5 1 edges at (34.2078, 13.35, 7) on bodies 41
extrude "Extrude24" add sketch "PCB" along normal blind 4.6 separate body contours A11 | A18 | A41 | A48 | A49 | L74 L75 L76 L77 makes body 42
extrude "Extrude25" add 1 faces at (32.3947, -3, 6.2) along direction (0, 0, 1) blind 4 draft -20 on bodies 42 bodies 42
draft "Draft1" angle 20 neutral plane through (36.928, -9, 1.6) pull (0, 1, 0) 1 faces at (34.176, -8.5147, 7.5333) on bodies 42
draft "Draft2" angle 20 neutral plane through (30.128, 9, 1.6) pull (0, -1, 0) 1 faces at (34.176, 8.5147, 7.5333) on bodies 42
extrude "Extrude26" cut sketch "PCB" against normal blind 0.5 from surface at 8.6 contours A11 | A18 | A41 | A48 | A49 bodies 42
move_face "OffsetFaces1" offset -0.8 5 faces at (33.356, -7.6113, 9.8667) (33.356, -4.1113, 9.8667) (33.356, -0.6113, 9.8667) (33.356, 2.8887, 9.8667) (33.356, 6.3887, 9.8667) on bodies 42
sketch "motor block" plane through (36.928, 0, 0) normal (1, 0, 0) x (0, 1, 0)
  line L0 (-9, 1.6) -> (9, 1.6)
  line L1 (9, 1.6) -> (9, 6.2)
  line L2 (9, 6.2) -> (-9, 6.2)
  line L3 (-9, 6.2) -> (-9, 1.6)
  line L4 (-8.5, 6) -> (-5.5, 6)
  line L5 (-5.5, 6) -> (-5.5, 1.8)
  line L6 (-5.5, 1.8) -> (-8.5, 1.8)
  line L7 (-8.5, 1.8) -> (-8.5, 6)
  line L8 (-5, 1.8) -> (-5, 6)
  line L9 (-5, 6) -> (-2, 6)
  line L10 (-2, 6) -> (-2, 1.8)
  line L11 (-2, 1.8) -> (-5, 1.8)
  line L12 (-1.5, 1.8) -> (-1.5, 6)
  line L13 (-1.5, 6) -> (1.5, 6)
  line L14 (1.5, 6) -> (1.5, 1.8)
  line L15 (1.5, 1.8) -> (-1.5, 1.8)
  line L16 (2, 1.8) -> (2, 6)
  line L17 (2, 6) -> (5, 6)
  line L18 (5, 6) -> (5, 1.8)
  line L19 (5, 1.8) -> (2, 1.8)
  line L20 (5.5, 1.8) -> (5.5, 6)
  line L21 (5.5, 6) -> (8.5, 6)
  line L22 (8.5, 6) -> (8.5, 1.8)
  line L23 (8.5, 1.8) -> (5.5, 1.8)
  circle A0 centre (-7, 3.3) radius 1
  circle A1 centre (-3.5, 3.3) radius 1
  circle A2 centre (0, 3.3) radius 1
  circle A3 centre (3.5, 3.3) radius 1
  circle A4 centre (7, 3.3) radius 1
  dimension "d219" = 0.5
  dimension "d220" = 0.2
  dimension "d221" = 0.2
  dimension "d224" = 3.5
  dimension "d225" = 0
  dimension "d226" = 3
  dimension "d227" = 2
  dimension "d230" = 3.5
  dimension "d231" = 0
  dimension "d276" = 1.5
  measures "d219" distance of L3 L7
  measures "d220" distance of L0 L6
  measures "d221" distance of L2 L4
  measures "d226" distance of L5.end L6.end
  measures "d227" diameter of A0
  measures "d276" distance of L6 A0.centre
extrude "Extrude27" cut sketch "motor block" against normal blind 1 contours L4 L5 L6 L7 | L8 L9 L10 L11 | L12 L13 L14 L15 | L16 L17 L18 L19 | L20 L21 L22 L23 | A0 | A1 | A2 | A3 | A4 bodies 42
extrude "Extrude28" cut sketch "motor block" against normal blind 1 from surface at -1 contours A0 | A1 | A2 | A3 | A4 bodies 42
extrude "Extrude29" add sketch "PCB" along normal blind 4.6 separate body contours A0 | A29 | A30 | A59 | A60 | L78 L79 L80 L81 makes body 43
extrude "Extrude30" add 1 faces at (26.621, 22.3782, 6.2) along direction (0, 0, 1) blind 4 draft -20 on bodies 43 bodies 43
draft "Draft3" angle 20 neutral plane through (32.4664, 19.7384, 1.6) pull (-0.707107, 0.707107, 0) 1 faces at (29.2608, 17.2191, 7.5333) on bodies 43
draft "Draft4" angle 20 neutral plane through (14.9301, 27.658, 1.6) pull (0.707107, -0.707107, 0) 1 faces at (17.2192, 29.2607, 7.5333) on bodies 43
sketch "drive block" plane through (26.1024, 26.1024, 0) normal (0.707107, 0.707107, 0) x (-0.707107, 0.707107, 0)
  line L0 (-9.0001, 1.6) -> (8.9999, 1.6)
  line L1 (8.9999, 1.6) -> (8.9999, 6.2)
  line L2 (8.9999, 6.2) -> (-9.0001, 6.2)
  line L3 (-9.0001, 6.2) -> (-9.0001, 1.6)
  line L4 (-8.5001, 5.7) -> (-5.5001, 5.7)
  line L5 (-5.5001, 5.7) -> (-5.5001, 2.1)
  line L6 (-5.5001, 2.1) -> (-8.5001, 2.1)
  line L7 (-8.5001, 2.1) -> (-8.5001, 5.7)
  line L8 (-2.0001, 5.7) -> (-2.0001, 2.1)
  line L9 (-2.0001, 2.1) -> (-5.0001, 2.1)
  line L10 (-5.0001, 2.1) -> (-5.0001, 5.7)
  line L11 (-5.0001, 5.7) -> (-2.0001, 5.7)
  line L12 (1.4999, 5.7) -> (1.4999, 2.1)
  line L13 (1.4999, 2.1) -> (-1.5001, 2.1)
  line L14 (-1.5001, 2.1) -> (-1.5001, 5.7)
  line L15 (-1.5001, 5.7) -> (1.4999, 5.7)
  line L16 (4.9999, 5.7) -> (4.9999, 2.1)
  line L17 (4.9999, 2.1) -> (1.9999, 2.1)
  line L18 (1.9999, 2.1) -> (1.9999, 5.7)
  line L19 (1.9999, 5.7) -> (4.9999, 5.7)
  line L20 (8.4999, 5.7) -> (8.4999, 2.1)
  line L21 (8.4999, 2.1) -> (5.4999, 2.1)
  line L22 (5.4999, 2.1) -> (5.4999, 5.7)
  line L23 (5.4999, 5.7) -> (8.4999, 5.7)
  circle A0 centre (-7.0001, 3.6) radius 1
  circle A1 centre (-3.5001, 3.6) radius 1
  circle A2 centre (-0.0001, 3.6) radius 1
  circle A3 centre (3.4999, 3.6) radius 1
  circle A4 centre (6.9999, 3.6) radius 1
  dimension "d253" = 0.5
  dimension "d254" = 0.5
  dimension "d255" = 0.5
  dimension "d256" = 3
  dimension "d259" = 3.5
  dimension "d260" = 0
  dimension "d261" = 2
  dimension "d262" = 1.5
  dimension "d265" = 3.5
  dimension "d266" = 0
  measures "d253" distance of L3 L7
  measures "d254" distance of L2 L4
  measures "d255" distance of L0 L6
  measures "d256" distance of L5.end L6.end
  measures "d261" diameter of A0
  measures "d262" distance of L6 A0.centre
extrude "Extrude31" cut sketch "drive block" against normal blind 1 contours L4 L5 L6 L7 | L8 L9 L10 L11 | L12 L13 L14 L15 | L16 L17 L18 L19 | L20 L21 L22 L23 | A0 | A1 | A2 | A3 | A4 bodies 43
extrude "Extrude32" cut sketch "drive block" against normal blind 1 from surface at -1 contours A0 | A1 | A2 | A3 | A4 bodies 43
extrude "Extrude33" cut sketch "PCB" against normal blind 0.5 from surface at 8.6 contours A0 | A29 | A30 | A59 | A60 bodies 43
move_face "OffsetFaces2" offset -0.8 5 faces at (28.5689, 18.1184, 9.8667) (25.588, 21.47, 10.0333) (23.6192, 23.0681, 9.8667) (21.1443, 25.543, 9.8667) (18.6695, 28.0178, 9.8667) on bodies 43
extrude "Extrude34" add sketch "PCB" along normal blind 4.6 separate body contours A12 | A13 | A17 | A43 | A46 | L82 L83 L84 L85 | L87 L88 L89 L90 makes body 44 at (20.815, -25.8422, 1.6) makes body 45 at (28.9089, -20.9539, 1.6)
extrude "Extrude35" add 1 faces at (20.815, -25.8422, 6.2) along direction (0, 0, 1) blind 4 draft -20 on bodies 44 bodies 44
extrude "Extrude36" add 1 faces at (28.9089, -20.9539, 6.2) along direction (0, 0, 1) blind 4 draft -20 on bodies 45 bodies 45
draft "Draft5" angle 20 neutral plane through (18.8351, -34.2332, 1.6) pull (0.707107, 0.707107, 0) 1 faces at (16.3159, -31.0277, 7.5333) on bodies 44
draft "Draft6" angle 20 neutral plane through (23.9355, -19.5161, 1.6) pull (0.707107, 0.707107, 0) 1 faces at (27.1411, -22.0354, 7.5333) on bodies 45
draft "Draft7" angle 20 neutral plane through (21.805, -21.6467, 1.6) pull (-0.707107, -0.707107, 0) 1 faces at (24.3242, -24.8523, 7.5333) on bodies 44
draft "Draft8" angle 20 neutral plane through (34.0472, -19.0211, 1.6) pull (-0.707107, -0.707107, 0) 1 faces at (30.8416, -16.5019, 7.5333) on bodies 45
extrude "Extrude37" cut sketch "PCB" against normal blind 0.5 from surface at 8.6 contours A12 | A13 | A17 | A43 | A46 bodies 44 45
move_face "OffsetFaces3" offset -0.8 5 faces at (17.7661, -31.045, 9.8667) (20.6097, -28.5051, 9.8667) (22.7159, -26.0952, 9.8667) (27.6749, -21.1362, 9.8667) (30.1498, -18.6613, 9.8667) on bodies 44 45
sketch "neo speaker" plane through (26.5342, -26.5342, 0) normal (0.707107, -0.707107, 0) x (0.707107, 0.707107, 0)
  line L0 (-10.8881, 1.6) -> (0.1119, 1.6)
  line L1 (0.1119, 1.6) -> (0.1119, 6.2)
  line L2 (0.1119, 6.2) -> (-10.8881, 6.2)
  line L3 (-10.8881, 6.2) -> (-10.8881, 1.6)
  line L4 (3.125, 1.6) -> (10.625, 1.6)
  line L5 (10.625, 1.6) -> (10.625, 6.2)
  line L6 (10.625, 6.2) -> (3.125, 6.2)
  line L7 (3.125, 6.2) -> (3.125, 1.6)
  line L8 (-10.3881, 5.7) -> (-7.3881, 5.7)
  line L9 (-7.3881, 5.7) -> (-7.3881, 2.1)
  line L10 (-7.3881, 2.1) -> (-10.3881, 2.1)
  line L11 (-10.3881, 2.1) -> (-10.3881, 5.7)
  line L12 (3.625, 5.7) -> (6.625, 5.7)
  line L13 (6.625, 5.7) -> (6.625, 2.1)
  line L14 (6.625, 2.1) -> (3.625, 2.1)
  line L15 (3.625, 2.1) -> (3.625, 5.7)
  line L16 (-3.8881, 2.1) -> (-6.8881, 2.1)
  line L17 (-6.8881, 2.1) -> (-6.8881, 5.7)
  line L18 (-6.8881, 5.7) -> (-3.8881, 5.7)
  line L19 (-3.8881, 5.7) -> (-3.8881, 2.1)
  line L20 (-0.3881, 2.1) -> (-3.3881, 2.1)
  line L21 (-3.3881, 2.1) -> (-3.3881, 5.7)
  line L22 (-3.3881, 5.7) -> (-0.3881, 5.7)
  line L23 (-0.3881, 5.7) -> (-0.3881, 2.1)
  line L24 (7.125, 2.1) -> (7.125, 5.7)
  line L25 (7.125, 5.7) -> (10.125, 5.7)
  line L26 (10.125, 5.7) -> (10.125, 2.1)
  line L27 (10.125, 2.1) -> (7.125, 2.1)
  circle A0 centre (-8.8881, 3.6) radius 1
  circle A1 centre (-5.3881, 3.6) radius 1
  circle A2 centre (-1.8881, 3.6) radius 1
  circle A3 centre (5.125, 3.6) radius 1
  circle A4 centre (8.625, 3.6) radius 1
  dimension "d305" = 0.5
  dimension "d306" = 0.5
  dimension "d307" = 0.5
  dimension "d308" = 0.5
  dimension "d309" = 0.5
  dimension "d310" = 0.5
  dimension "d311" = 3
  dimension "d312" = 3
  dimension "d315" = 3.5
  dimension "d316" = 0
  dimension "d319" = 3.5
  dimension "d320" = 0
  dimension "d321" = 2
  dimension "d322" = 2
  dimension "d325" = 3.5
  dimension "d326" = 0
  dimension "d327" = 2
  dimension "d328" = 2
  dimension "d331" = 3.5
  dimension "d332" = 0
  measures "d305" distance of L3 L11
  measures "d306" distance of L0 L10
  measures "d307" distance of L2 L8
  measures "d308" distance of L7 L15
  measures "d309" distance of L4 L14
  measures "d310" distance of L6 L12
  measures "d311" distance of L9.end L10.end
  measures "d312" distance of L13.end L14.end
  measures "d321" diameter of A0
  measures "d322" distance of L0 A0.centre
  measures "d327" diameter of A3
  measures "d328" distance of L4 A3.centre
extrude "Extrude38" cut sketch "neo speaker" against normal blind 1 contours L8 L9 L10 L11 | L12 L13 L14 L15 | L16 L17 L18 L19 | L20 L21 L22 L23 | L24 L25 L26 L27 | A0 | A1 | A2 | A3 | A4 bodies 44 45
extrude "Extrude39" cut sketch "neo speaker" against normal blind 1 from surface at -1 contours A0 | A1 | A2 | A3 | A4 bodies 44 45
extrude "Extrude40" add sketch "PCB" along normal blind 0.5 separate body contours A80 makes body 46
sketch "trim pot" plane through (0, 0, 2.1) normal (0, 0, 1) x (-1, 0, 0)
  circle A0 centre (-20.141, 20.194) radius 1.5
  line L0 (-19.891, 21.194) -> (-20.391, 21.194)
  line L1 (-20.391, 19.194) -> (-19.891, 19.194)
  line L2 (-19.141, 20.444) -> (-19.141, 19.944)
  line L3 (-21.141, 19.944) -> (-21.141, 20.444)
  line L4 (-19.891, 20.444) -> (-19.141, 20.444)
  line L5 (-19.891, 19.194) -> (-19.891, 19.944)
  line L6 (-19.891, 20.444) -> (-19.891, 21.194)
  line L7 (-19.141, 19.944) -> (-19.891, 19.944)
  line L8 (-20.391, 19.944) -> (-21.141, 19.944)
  line L9 (-21.141, 20.444) -> (-20.391, 20.444)
  line L10 (-20.391, 21.194) -> (-20.391, 20.444)
  line L11 (-20.391, 19.944) -> (-20.391, 19.194)
  point P0 (-20.141, 20.194)
  point P1 (-20.141, 20.194)
  dimension "d343" = 2
  dimension "d344" = 0.5
  dimension "d345" = 2
  dimension "d346" = 0.5
  measures "d343" distance of L0.end L1.start
  measures "d344" distance of L1.start L1.end
  measures "d345" distance of L2.end L3.start
  measures "d346" distance of L2.start L2.end
extrude "Extrude41" cut sketch "trim pot" against normal blind 0.2 contours L0 L1 L2 L3 L4 L5 L6 L7 L8 L9 L10 L11 bodies 46
extrude "Extrude42" add sketch "PCB" along normal blind 0.6 separate body contours L91 L92 L93 L94 makes body 47
extrude "Extrude43" add sketch "PCB" along normal blind 0.5 separate body contours L97 L98 L99 L100 makes body 48
move_body "Move1" bodies 48 to x (1, 0, 0) y (0, 1, 0) z (0, 0, 1) at (-1.3, -1.2, 0)
extrude "Extrude44" add sketch "PCB" along normal blind 1 separate body contours L103 L104 L105 L106 makes body 49
move_body "Move2" bodies 49 to x (1, 0, 0) y (0, 1, 0) z (0, 0, 1) at (-2, -2, 0)
component "servo block" placed x (1, 0, 0) y (0, 1, 0) z (0, 0, 1) at (0, 0, 0)
equation "d2 = ( 81.28 / 2 ) * 1 mm"
equation "d91 = ( 2.54 / 2 ) * 1 mm"
equation "d134 = ( 9 / 2 ) * 1 mm"
named bodies: "PCB", "SIO block", "microUSB", "neopixel", "DC Jack", "reset", "switch", "LED bad", "LED OK", "cap1", "cap2", "motor block", "drive block", "neopixel block", "speaker block", "trim pot", "samd21", "htssop", "so16"
